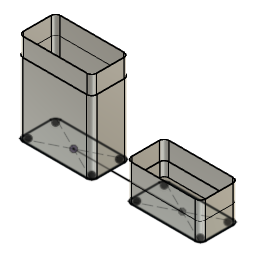
parametric_design_2 (Autodesk Fusion 360 design; units mm, degrees)
part number: 2025-09-04-15-13-34-922
Autodesk Fusion 360 part; units mm, degrees
sketch "Sketch1" plane through (0, 0, 0) normal (0, 0, 1) x (1, 0, 0)
  line L0 (22, -12.5) -> (-22, -12.5)
  line L1 (-25, -9.5) -> (-25, 9.5)
  line L2 (-22, 12.5) -> (22, 12.5)
  line L3 (25, 9.5) -> (25, -9.5)
  line L4 (25, -12.5) -> (-25, 12.5) construction
  line L5 (-25, -12.5) -> (25, 12.5) construction
  line L6 (0, 0) -> (75, 0)
  line L7 (97, -12.5) -> (53, -12.5)
  line L8 (50, -9.5) -> (50, 9.5)
  line L9 (53, 12.5) -> (97, 12.5)
  line L10 (100, 9.5) -> (100, -9.5)
  line L11 (100, -12.5) -> (50, 12.5) construction
  line L12 (50, -12.5) -> (100, 12.5) construction
  arc A0 (53, 12.5) -> (50, 9.5) centre (53, 9.5) ccw
  arc A1 (100, 9.5) -> (97, 12.5) centre (97, 9.5) ccw
  arc A2 (50, -9.5) -> (53, -12.5) centre (53, -9.5) ccw
  arc A3 (97, -12.5) -> (100, -9.5) centre (97, -9.5) ccw
  arc A4 (50, -9.5) -> (53, -12.5) centre (53, -9.5) ccw
  arc A5 (-22, 12.5) -> (-25, 9.5) centre (-22, 9.5) ccw
  arc A6 (-25, -9.5) -> (-22, -12.5) centre (-22, -9.5) ccw
  arc A7 (25, 9.5) -> (22, 12.5) centre (22, 9.5) ccw
  arc A8 (22, -12.5) -> (25, -9.5) centre (22, -9.5) ccw
  arc A9 (25, 9.5) -> (22, 12.5) centre (22, 9.5) ccw
  arc A10 (-25, -9.5) -> (-22, -12.5) centre (-22, -9.5) ccw
  arc A11 (22, -12.5) -> (25, -9.5) centre (22, -9.5) ccw
  arc A12 (25.3, 9.5) -> (22, 12.8) centre (22, 9.5) ccw
  line L13 (-22, 12.8) -> (22, 12.8)
  arc A13 (-22, 12.8) -> (-25.3, 9.5) centre (-22, 9.5) ccw
  line L14 (-25.3, -9.5) -> (-25.3, 9.5)
  arc A14 (-25.3, -9.5) -> (-22, -12.8) centre (-22, -9.5) ccw
  line L15 (22, -12.8) -> (-22, -12.8)
  arc A15 (22, -12.8) -> (25.3, -9.5) centre (22, -9.5) ccw
  line L16 (25.3, 9.5) -> (25.3, -9.5)
  arc A16 (25.6, 9.5) -> (22, 13.1) centre (22, 9.5) ccw
  line L17 (-22, 13.1) -> (22, 13.1)
  arc A17 (-22, 13.1) -> (-25.6, 9.5) centre (-22, 9.5) ccw
  line L18 (-25.6, -9.5) -> (-25.6, 9.5)
  arc A18 (-25.6, -9.5) -> (-22, -13.1) centre (-22, -9.5) ccw
  line L19 (22, -13.1) -> (-22, -13.1)
  arc A19 (22, -13.1) -> (25.6, -9.5) centre (22, -9.5) ccw
  line L20 (25.6, 9.5) -> (25.6, -9.5)
  arc A20 (100.3, 9.5) -> (97, 12.8) centre (97, 9.5) ccw
  line L21 (53, 12.8) -> (97, 12.8)
  arc A21 (53, 12.8) -> (49.7, 9.5) centre (53, 9.5) ccw
  line L22 (49.7, -9.5) -> (49.7, 9.5)
  arc A22 (49.7, -9.5) -> (53, -12.8) centre (53, -9.5) ccw
  line L23 (97, -12.8) -> (53, -12.8)
  arc A23 (97, -12.8) -> (100.3, -9.5) centre (97, -9.5) ccw
  line L24 (100.3, 9.5) -> (100.3, -9.5)
  arc A24 (100.6, 9.5) -> (97, 13.1) centre (97, 9.5) ccw
  line L25 (53, 13.1) -> (97, 13.1)
  arc A25 (53, 13.1) -> (49.4, 9.5) centre (53, 9.5) ccw
  line L26 (49.4, -9.5) -> (49.4, 9.5)
  arc A26 (49.4, -9.5) -> (53, -13.1) centre (53, -9.5) ccw
  line L27 (97, -13.1) -> (53, -13.1)
  arc A27 (97, -13.1) -> (100.6, -9.5) centre (97, -9.5) ccw
  line L28 (100.6, 9.5) -> (100.6, -9.5)
  point P0 (75, 0)
  dimension "d9" = 50
  dimension "d10" = 25
  dimension "d12" = 75
  dimension "d13" = 50
  dimension "d14" = 25
  dimension "d16" = 3
  dimension "d17" = 3
  dimension "d18" = 3
  dimension "d19" = 3
  dimension "d20" = 3
  dimension "d21" = 3
  dimension "d22" = 3
  dimension "d23" = 3
  constraint horizontal L0
  constraint perpendicular L0 L1
  constraint parallel L0 L2
  constraint parallel L1 L3
  constraint coincident L4 L6.start
  constraint coincident L5 L6.start
  constraint coincident L6.start origin
  constraint parallel L2 L6
  constraint horizontal L7
  constraint perpendicular L7 L8
  constraint parallel L7 L9
  constraint parallel L8 L10
  constraint coincident L11 P0
  constraint coincident L12 P0
  constraint coincident P0 L6.end
  constraint coincident L11.end L9
  constraint coincident L11.end L8
  constraint tangent L9 A0
  constraint tangent L8 A0
  constraint coincident L12.end L9
  constraint coincident L12.end L10
  constraint tangent L9 A1
  constraint tangent L10 A1
  constraint coincident L12.start L7
  constraint coincident L12.start L8
  constraint tangent L7 A2
  constraint tangent L8 A2
  constraint equal A1 A2
  constraint coincident L11.start L7
  constraint coincident L11.start L10
  constraint tangent L7 A3
  constraint tangent L10 A3
  constraint coincident L7 A2.end
  constraint coincident L8 A2.start
  constraint tangent L7 A4
  constraint tangent L8 A4
  constraint coincident L4.end L2
  constraint coincident L4.end L1
  constraint tangent L2 A5
  constraint tangent L1 A5
  constraint coincident L5.start L1
  constraint coincident L5.start L0
  constraint tangent L1 A6
  constraint tangent L0 A6
  constraint equal A5 A6
  constraint coincident L5.end L3
  constraint coincident L5.end L2
  constraint tangent L3 A7
  constraint tangent L2 A7
  constraint equal A5 A7
  constraint coincident L4.start L0
  constraint coincident L4.start L3
  constraint tangent L0 A8
  constraint tangent L3 A8
  constraint equal A5 A8
  constraint coincident L2 A7.end
  constraint coincident L3 A7.start
  constraint tangent L2 A9
  constraint tangent L3 A9
  constraint coincident L0 A6.end
  constraint coincident L1 A6.start
  constraint tangent L0 A10
  constraint tangent L1 A10
  constraint coincident L0 A8.start
  constraint coincident L3 A8.end
  constraint tangent L0 A11
  constraint tangent L3 A11
  measures "d9" distance of L4.end L5.end
  measures "d10" distance of L5.start L4.end
  measures "d12" distance of L6.start P0
  measures "d13" distance of L11.end L12.end
  measures "d14" distance of L12.start L11.end
  measures "d16" radius of A0
  measures "d17" radius of A1
  measures "d18" radius of A3
  measures "d19" radius of A4
  measures "d20" radius of A5
  measures "d21" radius of A9
  measures "d22" radius of A10
  measures "d23" radius of A11
extrude "Extrude1" add sketch "Sketch1" along normal blind 3 contours L7 L8 L9 L10 A0 A1 A2 A3 A4 makes body 1
extrude "Extrude2" add sketch "Sketch1" along normal up to surface (3 mm away) separate body contours L0 L1 L2 L3 A5 A6 A7 A8 A9 A10 A11 makes body 2
extrude "Extrude3" add sketch "Sketch1" along normal blind 50 separate body contours A16 L17 A17 L18 A18 L19 A19 L20 makes body 3
extrude "Extrude4" add sketch "Sketch1" along normal blind 62.5 contours A12 L13 A13 L14 A14 L15 A15 L16 bodies 2 3
extrude "Extrude5" add sketch "Sketch1" along normal blind 25 separate body contours A24 L25 A25 L26 A26 L27 A27 L28 makes body 4
extrude "Extrude6" add sketch "Sketch1" along normal blind 12.5 contours A20 L21 A21 L22 A22 L23 A23 L24 bodies 1 4
equation "RECLONG = 50 mm"
equation "recShort = RECLONG / 2"
equation "FILLET = 3 mm"
equation "RECLENGTH = 50 mm"
equation "cupLength = RECLENGTH + RECLENGTH / 4"
equation "tipLength = RECLENGTH / 2"
equation "tipInlength = cupLength - RECLENGTH"
equation "d9 = RECLONG"
equation "d10 = recShort"
equation "distance = RECLONG * 1.5"
equation "d12 = distance"
equation "d13 = RECLONG"
equation "d14 = recShort"
equation "snugslipoffset = 0.3 mm"
equation "d16 = FILLET"
equation "d17 = FILLET"
equation "d18 = FILLET"
equation "d19 = FILLET"
equation "d20 = FILLET"
equation "d21 = FILLET"
equation "d22 = FILLET"
equation "d23 = FILLET"
equation "d24 = -snugslipoffset"
equation "d25 = -snugslipoffset"
equation "d26 = -snugslipoffset"
equation "d27 = -snugslipoffset"
equation "d32 = RECLENGTH"
equation "d34 = cupLength"
equation "d36 = tipLength"
equation "d38 = tipInlength"
